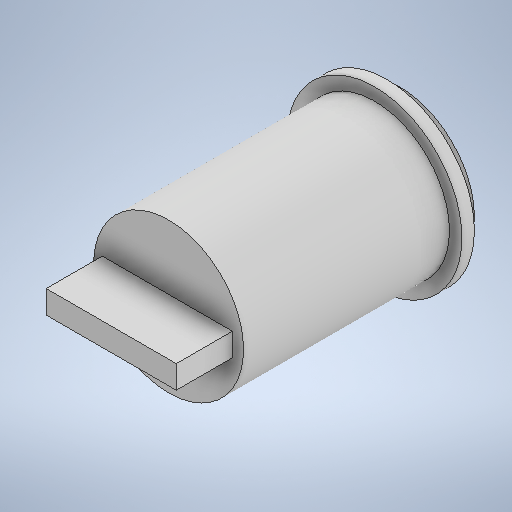
# Autodesk Inventor part: Knopf
Saved by Autodesk Inventor 2025.1 (Build 291241000, 241)
## iProperties
Created: 2025-02-01
Part Number: Knopf
Material: Generisch
Document SubType Name: Modeling
Designer: joebe
Density: 1 g/cm^3
Appearance: Vorgabe
Author: joebe
Autodesk Inventor part; units mm, degrees
ref_plane "YZ Plane" through (0, 0, 0) normal (1, 0, 0) x (0, 1, 0)
ref_plane "XZ Plane" through (0, 0, 0) normal (0, 1, 0) x (-1, 0, 0)
ref_plane "XY Plane" through (0, 0, 0) normal (0, 0, 1) x (1, 0, 0)
sketch "Skizze1" plane through (0, 0, 0) normal (0, 0, 1) x (1, 0, 0)
  line L0 (0, 0) -> (6, 0)
  line L1 (6, 0) -> (6, 16.5)
  line L2 (6, 16.5) -> (7, 16.5)
  line L3 (7, 16.5) -> (7, 17.5)
  line L4 (7, 17.5) -> (5.8187, 17.8052)
  line L5 (5.8187, 17.8052) -> (5.9982, 18.5)
  line L6 (5.9982, 18.5) -> (0, 18.5)
  line L7 (0, 18.5) -> (0, 0)
  point P0 (6.5, 16.5)
  dimension "d0" = 6
  dimension "d1" = 16.5
  dimension "d2" = 7
  dimension "d3" = 1
  dimension "d4" = 2
  constraints: 16 end point, 5 perpendicular, 1 horizontal, 1 midpoint, 1 parallel
  measures "d0" distance between parallel lines of L7 L1
  measures "d1" distance of L0.end L1.end
  measures "d2" distance between parallel lines of L7 L3
  measures "d3" distance of L2.end L3.end
  measures "d4" distance from line of point (6.5, 16.5) L6
revolve "Umdrehung1" add sketch "Skizze1" angle 360 about axis through (0, 18.5, 0) along (0, -1, 0)
sketch "Skizze2" plane through (0, 0, 0) normal (0, -1, 0) x (1, 0, 0)
  line L0 (-5.3128, 0.8351) -> (5.1112, 0.8351)
  line L1 (5.1112, 0.8351) -> (5.1112, -1.0078)
  line L2 (5.1112, -1.0078) -> (-5.3128, -1.0078)
  line L3 (-5.3128, -1.0078) -> (-5.3128, 0.8351)
  point P0 (0, 0)
  constraints: 8 end point, 2 parallel, 1 horizontal, 1 perpendicular
extrude "Extrusion1" add sketch "Skizze2" along normal blind 4.5
